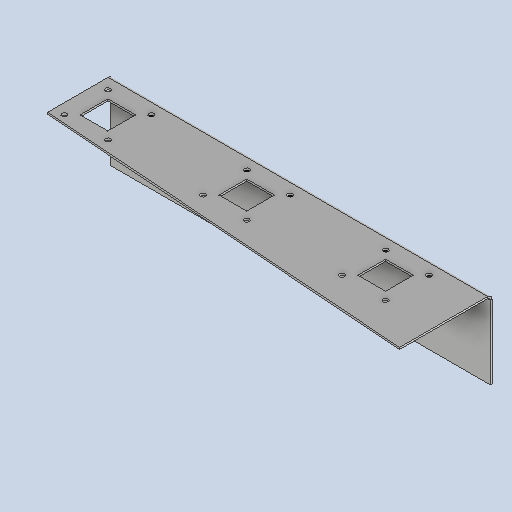
# Autodesk Inventor part: ANP 1422 BOTTOM FDS diameter way up
Saved by Autodesk Inventor 2025 (Build 290162010, 162A)
## iProperties
Created: 2024-12-09
Part Number: ANP 1422 BOTTOM FDS diameter way up
Material: Stainless Steel
Document SubType Name: Sheet Metal
Designer: user
Mass: 3269.02 g
Surface Area: 1007.63 cm^2
Volume: 408.627 cm^3
Density: 8 g/cm^3
Flat Pattern Width: 18.0202 cm
Flat Pattern Length: 41 cm
Flat Pattern Area: 738.828 cm^2
Sheet Metal Rule: AISI304 2mm Die16
Sheet Metal Width: 180,202 mm
Sheet Metal Length: 410,000 mm
Sheet Metal Area: 73882,816 mm^2
Appearance: Default
Main_way_hight: 100,000 mm
Main_way_lenth: 410,000 mm
Small_ways_cross_H: 30,000 mm
Small_ways_cross_W: 30,000 mm
Author: user
Autodesk Inventor part; units mm, degrees
ref_plane "YZ Plane" through (0, 0, 0) normal (1, 0, 0) x (0, 1, 0)
ref_plane "XZ Plane" through (0, 0, 0) normal (0, 1, 0) x (-1, 0, 0)
ref_plane "XY Plane" through (0, 0, 0) normal (0, 0, 1) x (1, 0, 0)
sketch "Sketch1" plane through (0, 0, 0) normal (0, 0, 1) x (1, 0, 0)
  line L0 (0, 0) -> (-410, 0)
  line L1 (0, -100) -> (0, 0)
  line L2 (-410, 0) -> (-410, -70)
  line L3 (-410, -70) -> (0, -100)
  point P0 (0, -50)
  dimension "d32" = 100
  dimension "d60" = 70
  dimension "d61" = 410
  measures "d32" distance of L1.start L0.start
  measures "d60" distance of L0.end L2.end
  measures "d61" distance between parallel lines of L1 L2
extrude "Plate1" add sketch "Sketch1" along normal blind 2
sketch "Sketch8" plane through (0, 0, 2) normal (0, 0, 1) x (1, 0, 0)
  line L0 (-60, -55) -> (-90, -55)
  line L1 (-90, -55) -> (-90, -25)
  line L2 (-90, -25) -> (-60, -25)
  line L3 (-60, -25) -> (-60, -55)
  line L4 (-60, -55) -> (-90, -25) construction
  line L5 (-90, -55) -> (-60, -25) construction
  circle A0 centre (-51.5147, -63.4853) radius 2.75
  circle A1 centre (-98.4853, -63.4853) radius 2.75
  circle A2 centre (-98.4853, -16.5147) radius 2.75
  circle A3 centre (-51.5147, -16.5147) radius 2.75
  circle A4 centre (-75, -40) radius 33.2132 construction
  line L6 (0, 0) -> (0, -100) projected
  line L7 (-410, 0) -> (0, 0) projected
  line L8 (-90, -55) -> (-98.4853, -63.4853) construction
  dimension "d51" = 30
  dimension "d52" = 30
  dimension "d53" = 5.5
  dimension "d72" = 75
  dimension "d73" = 40
  dimension "d74" = 12
  constraints: 14 end point, 5 centre point, 4 point on circle, 4 point on line, 3 equal radius, 2 midpoint, 2 parallel, 1 coincident, 1 horizontal, 1 perpendicular
  measures "d51" distance of L0.start L0.end
  measures "d52" distance of L0.end L1.end
  measures "d53" diameter of A0
  measures "d72" distance from line of L6 point (-75, -40)
  measures "d73" distance from line of point (-75, -40) L7
  measures "d74" distance of L8.end L0.end
extrude "Cut3" cut sketch "Sketch8" against normal blind 2
pattern_linear "Rectangular Pattern1" count 3 spacing 150 along (-1, 0, 0) of "Cut3"
sketch "Sketch9" plane through (0, -2, 2) normal (0, 1, 0) x (-1, 0, 0)
  line L0 (410, 0) -> (0, 0)
  line L1 (0, 0) -> (0, -84)
  line L2 (0, -84) -> (410, -84)
  line L3 (410, -84) -> (410, 0)
  constraints: 6 end point, 1 horizontal, 1 perpendicular, 1 vertical
edge flange "Flange3" height 84 angle 90 thickness 2 bend radius 2.75 thickness toward (0, 1, 0) relief round relief width 2 relief depth 1 edges at (-205, 0, 0) wall of the first edge with corners at (-410, -2, 2) (0, -2, 2) (0, -2, -82) (-410, -2, -82)
bend "Bend3"
corner "Corner3"
equation "\"d32\" = Main_way_hight"
equation "\"d61\" = Main_way_lenth"
equation "\"d51\" = Small_ways_cross_W"
equation "\"d52\" = Small_ways_cross_H"
equation "\"d55\" = Thickness"
equation "\"d2\" = Thickness"
equation "\"d62\" = BendReliefWidth"
equation "\"d63\" = BendReliefDepth"
equation "\"d64\" = MinimumRemnant"
equation "\"d65\" = TransitionRadius"
equation "\"d66\" = MAIN_7_central_window_width + 2 * Thickness"
equation "\"d68\" = BendRadius"
equation "\"d69\" = CornerReliefSize"
equation "\"d70\" = GapSize"
equation "\"d71\" = JacobiRadiusSize"
equation "\"BendReliefWidth\" = Thickness"
equation "\"BendReliefDepth\" = 0.5 * Thickness"
equation "\"CornerReliefSize\" = 4 * Thickness"
equation "\"MinimumRemnant\" = 2 * Thickness"
equation "\"TransitionRadius\" = BendRadius"
equation "\"JacobiRadiusSize\" = BendRadius"
equation "\"GapSize\" = Thickness"
equation "\"Main_way_hight\" = 100"
equation "\"Main_way_lenth\" = 410"
equation "\"Small_ways_cross_H\" = 30"
equation "\"Small_ways_cross_W\" = Small_ways_cross_H"
equation "\"Thickness\" = 2"
equation "\"MAIN_7_central_window_width\" = 80"
equation "\"BendRadius\" = 2.75"
body "Solid1"
